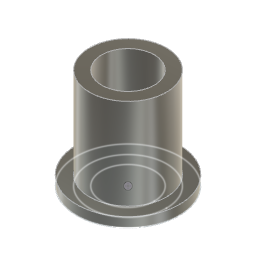
ECS Bleed Air Shaft Spacer v2 (Autodesk Fusion 360 design; units mm, degrees)
Autodesk Fusion 360 part; units mm, degrees
sketch "Sketch1" plane through (0, 0, 0) normal (0, 0, 1) x (1, 0, 0)
  circle A0 centre (0, 0) radius 3.25
  circle A1 centre (0, 0) radius 4.75
  circle A2 centre (0, 0) radius 6.35
  dimension "d1" = 6.5
  dimension "d2" = 9.5
  dimension "d3" = 12.7
  constraint coincident A0.centre A1.centre
  constraint concentric A0 A1
  constraint concentric A0 A2
  measures "d1" diameter of A0
  measures "d2" diameter of A1
  measures "d3" diameter of A2
extrude "Extrude1" add sketch "Sketch1" along normal blind 1.2 contours A2
extrude "Extrude2" add sketch "Sketch1" along normal blind 13.6 contours A1
extrude "Extrude3" cut 1 faces at (4.2202, -0.3974, 13.6) along direction (0, 0, -1) blind 1.2
named bodies: "ECS Bleed Air Shaft Support"
